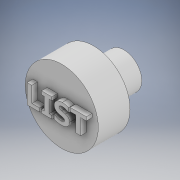
# Autodesk Inventor part: IPC List key
Saved by Autodesk Inventor 2022 (Build 260153000, 153)
## iProperties
Created: 2022-01-01
Part Number: IPC List key
Material: Generic
Document SubType Name: Modeling
Designer: solor
Density: 1 g/cm^3
Appearance: Default
Author: solor
Autodesk Inventor part; units mm, degrees
ref_plane "YZ Plane" through (0, 0, 0) normal (1, 0, 0) x (0, 1, 0)
ref_plane "XZ Plane" through (0, 0, 0) normal (0, 1, 0) x (-1, 0, 0)
ref_plane "XY Plane" through (0, 0, 0) normal (0, 0, 1) x (1, 0, 0)
sketch "Sketch1" plane through (0, 0, 0) normal (0, 0, 1) x (1, 0, 0)
  circle A0 centre (0, 0) radius 6.22 construction
  circle A1 centre (0, 0) radius 2.8
  line L0 (-0.675, 0.675) -> (-0.675, 2.025)
  line L1 (-0.675, 2.025) -> (0.675, 2.025)
  line L2 (0.675, 2.025) -> (0.675, 0.675)
  line L3 (0.675, 0.675) -> (2.025, 0.675)
  line L4 (2.025, 0.675) -> (2.025, -0.675)
  line L5 (2.025, -0.675) -> (0.675, -0.675)
  line L6 (0.675, -0.675) -> (0.675, -2.025)
  line L7 (0.675, -2.025) -> (-0.675, -2.025)
  line L8 (-0.675, -2.025) -> (-0.675, -0.675)
  line L9 (-0.675, -0.675) -> (-2.025, -0.675)
  line L10 (-2.025, -0.675) -> (-2.025, 0.675)
  line L11 (-2.025, 0.675) -> (-0.675, 0.675)
  circle A2 centre (0, 0) radius 5.75
  point P0 (-6.07, -6.1)
  dimension "d0" = 12.44
  dimension "d1" = 0.47
  constraints: 24 end point, 3 centre point, 1 coincident
  measures "d0" diameter of A0
  measures "d1" radial gap between concentric circles of A0 A2
extrude "Extrusion1" add sketch "Sketch1" along normal blind 5 contours A1 | L0 L1 L2 L3 L4 L5 L6 L7 L8 L9 L10 L11 | A2
extrude "Extrusion2" add sketch "Sketch1" against normal blind 4.8 contours A1
sketch "Sketch2" plane through (0, 0, 5) normal (0, 0, 1) x (1, 0, 0)
  point P0 (0, 0)
sketch "Sketch3" plane through (0, 0, 5) normal (0, 0, 1) x (1, 0, 0)
  line L0 (-4.8809, 1.4783) -> (4.8809, 1.4783) construction
  line L1 (4.8809, 1.4783) -> (4.8809, -1.6654) construction
  line L2 (4.8809, -1.6654) -> (-4.8809, -1.6654) construction
  line L3 (-4.8809, -1.6654) -> (-4.8809, 1.4783) construction
  line L4 (-2.5303, -1.6261) -> (-4.5645, -1.6261)
  line L5 (-4.5645, -1.6261) -> (-4.5645, 1.4239)
  line L6 (-4.5645, 1.4239) -> (-3.7983, 1.4239)
  line L7 (-3.7983, 1.4239) -> (-3.7983, -1.0452)
  line L8 (-3.7983, -1.0452) -> (-2.5303, -1.0452)
  line L9 (-2.5303, -1.0452) -> (-2.5303, -1.6261)
  line L10 (-0.6469, -1.6261) -> (-2.2881, -1.6261)
  line L11 (-2.2881, -1.6261) -> (-2.2881, -1.0947)
  line L12 (-2.2881, -1.0947) -> (-1.8506, -1.0947)
  line L13 (-1.8506, -1.0947) -> (-1.8506, 0.8925)
  line L14 (-1.8506, 0.8925) -> (-2.2881, 0.8925)
  line L15 (-2.2881, 0.8925) -> (-2.2881, 1.4239)
  line L16 (-2.2881, 1.4239) -> (-0.6469, 1.4239)
  line L17 (-0.6469, 1.4239) -> (-0.6469, 0.8925)
  line L18 (-0.6469, 0.8925) -> (-1.0844, 0.8925)
  line L19 (-1.0844, 0.8925) -> (-1.0844, -1.0947)
  line L20 (-1.0844, -1.0947) -> (-0.6469, -1.0947)
  line L21 (-0.6469, -1.0947) -> (-0.6469, -1.6261)
  spline S0 degree 2 poles (0.8039, -1.6804) (0.4529, -1.6804) (-0.076, -1.5445) (-0.3034, -1.4456) knots 0 0 0 1 2 2 2
  line L22 (-0.3034, -1.4456) -> (-0.3034, -0.719)
  line L23 (-0.3034, -0.719) -> (-0.2342, -0.719)
  spline S1 degree 2 poles (-0.2342, -0.719) (-0.0043, -0.9142) (0.5469, -1.1243) (0.8064, -1.1243) knots 0 0 0 1 2 2 2
  spline S2 degree 2 poles (0.8064, -1.1243) (0.8731, -1.1243) (1.0882, -1.0947) (1.1524, -1.065) knots 0 0 0 1 2 2 2
  spline S3 degree 2 poles (1.1524, -1.065) (1.2315, -1.0304) (1.3427, -0.9044) (1.3427, -0.803) knots 0 0 0 1 2 2 2
  spline S4 degree 2 poles (1.3427, -0.803) (1.3427, -0.6868) (1.1623, -0.5435) (1.0387, -0.5114) knots 0 0 0 1 2 2 2
  spline S5 degree 2 poles (1.0387, -0.5114) (0.883, -0.4693) (0.5296, -0.3977) (0.3738, -0.3433) knots 0 0 0 1 2 2 2
  spline S6 degree 2 poles (0.3738, -0.3433) (0.0204, -0.2197) (-0.2861, 0.2029) (-0.2861, 0.5193) knots 0 0 0 1 2 2 2
  spline S7 degree 2 poles (-0.2861, 0.5193) (-0.2861, 0.9469) (0.4381, 1.4783) (0.9819, 1.4783) knots 0 0 0 1 2 2 2
  spline S8 degree 2 poles (0.9819, 1.4783) (1.2538, 1.4783) (1.7926, 1.3671) (2.0051, 1.2732) knots 0 0 0 1 2 2 2
  line L24 (2.0051, 1.2732) -> (2.0051, 0.5762)
  line L25 (2.0051, 0.5762) -> (1.9384, 0.5762)
  spline S9 degree 2 poles (1.9384, 0.5762) (1.7679, 0.722) (1.2785, 0.9222) (1.0214, 0.9222) knots 0 0 0 1 2 2 2
  spline S10 degree 2 poles (1.0214, 0.9222) (0.9201, 0.9222) (0.7619, 0.8925) (0.6729, 0.853) knots 0 0 0 1 2 2 2
  spline S11 degree 2 poles (0.6729, 0.853) (0.6012, 0.8209) (0.4974, 0.6923) (0.4974, 0.6132) knots 0 0 0 1 2 2 2
  spline S12 degree 2 poles (0.4974, 0.6132) (0.4974, 0.4946) (0.663, 0.3587) (0.9003, 0.3043) knots 0 0 0 1 2 2 2
  spline S13 degree 2 poles (0.9003, 0.3043) (1.0535, 0.2697) (1.3378, 0.2029) (1.5009, 0.1461) knots 0 0 0 1 2 2 2
  spline S14 degree 2 poles (1.5009, 0.1461) (1.8173, 0.0299) (2.1262, -0.3556) (2.1262, -0.672) knots 0 0 0 1 2 2 2
  spline S15 degree 2 poles (2.1262, -0.672) (2.1262, -1.1268) (1.4119, -1.6804) (0.8039, -1.6804) knots 0 0 0 1 2 2 2
  line L26 (3.105, -1.6261) -> (3.105, 0.8431)
  line L27 (3.105, 0.8431) -> (2.2029, 0.8431)
  line L28 (2.2029, 0.8431) -> (2.2029, 1.4239)
  line L29 (2.2029, 1.4239) -> (4.7734, 1.4239)
  line L30 (4.7734, 1.4239) -> (4.7734, 0.8431)
  line L31 (4.7734, 0.8431) -> (3.8712, 0.8431)
  line L32 (3.8712, 0.8431) -> (3.8712, -1.6261)
  line L33 (3.8712, -1.6261) -> (3.105, -1.6261)
  point P0 (0, -1.6654)
  point P1 (0, 0)
  point P2 (0, 0)
  constraints: 1 midpoint, 2 other
extrude "Extrusion5" add sketch "Sketch3" along normal blind 0.9
body "Solid1"
